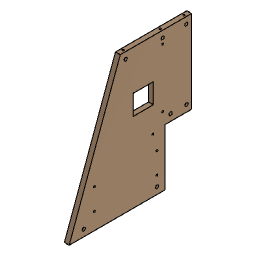
Side Panel Right (Autodesk Fusion 360 design; units mm, degrees)
Autodesk Fusion 360 part; units mm, degrees
sketch "Right" plane through (0, 0, 0) normal (1, 0, 0) x (0, 1, 0)
  line L0 (0, 0) -> (360, 0)
  line L1 (460, 212.5) -> (460, 524)
  line L2 (460, 524) -> (192, 524)
  line L3 (360, 0) -> (360, 212.5)
  line L4 (360, 212.5) -> (460, 212.5)
  line L5 (192, 524) -> (0, 0)
  line L6 (241, 374) -> (316, 374)
  line L7 (316, 374) -> (316, 299)
  line L8 (316, 299) -> (241, 299)
  line L9 (241, 299) -> (241, 374)
  line L10 (460, 499) -> (182.8397, 499) construction
  line L11 (460, 237.5) -> (316, 237.5) construction
  line L12 (360, 25) -> (9.1603, 25) construction
  line L13 (351, 524) -> (351, 250) construction
  circle A0 centre (351, 499) radius 6
  circle A1 centre (212, 499) radius 6
  circle A2 centre (440, 499) radius 6
  circle A3 centre (351, 479) radius 3.5
  circle A4 centre (351, 259) radius 3.5
  circle A5 centre (441, 237.5) radius 6
  circle A6 centre (381, 237.5) radius 6
  line L14 (330, 0) -> (330, 175) construction
  line L15 (330, 63) -> (95, 63) construction
  line L16 (95, 63) -> (95, 143) construction
  line L17 (95, 143) -> (330, 143) construction
  line L18 (330, 143) -> (330, 63) construction
  circle A7 centre (330, 63) radius 3.5
  circle A8 centre (330, 143) radius 3.5
  circle A9 centre (95, 143) radius 3.5
  circle A10 centre (95, 63) radius 3.5
  circle A11 centre (330, 25) radius 6
  circle A12 centre (55, 25) radius 6
  circle A13 centre (315, 204) radius 3.5
  dimension "d6" = 212.5
  dimension "d7" = 100
  dimension "d8" = 360
  dimension "d9" = 268
  dimension "d10" = 524
  dimension "d11" = 75
  dimension "d12" = 75
  dimension "d13" = 150
  dimension "d14" = 144
  dimension "d15" = 25
  dimension "d16" = 25
  dimension "d17" = 25
  dimension "d18" = 109
  dimension "d19" = 12
  dimension "d20" = 12
  dimension "d21" = 12
  dimension "d22" = 7
  dimension "d23" = 7
  dimension "d24" = 12
  dimension "d25" = 12
  dimension "d26" = 30
  dimension "d27" = 80
  dimension "d28" = 235
  dimension "d29" = 7
  dimension "d30" = 7
  dimension "d31" = 7
  dimension "d32" = 7
  dimension "d33" = 12
  dimension "d34" = 12
  dimension "d35" = 275
  dimension "d36" = 63
  dimension "d37" = 7
  dimension "d38" = 55
  dimension "d39" = 36
  dimension "d40" = 60
  dimension "d41" = 19
  dimension "d42" = 89
  dimension "d43" = 20
  dimension "d44" = 139
  dimension "d45" = 20
  dimension "d46" = 220
  constraint horizontal L0
  constraint vertical L1
  constraint horizontal L2
  constraint coincident L0.start L5.end
  constraint vertical L3
  constraint horizontal L4
  constraint horizontal L6
  constraint vertical L7
  constraint horizontal L8
  constraint vertical L9
  constraint coincident L1 L10.start
  constraint coincident L5 L10.end
  constraint perpendicular L1 L10
  constraint coincident L1 L11.start
  constraint perpendicular L1 L11
  constraint coincident L3 L12.start
  constraint coincident L5 L12.end
  constraint perpendicular L3 L12
  constraint coincident L2 L13.start
  constraint perpendicular L10 L13
  constraint coincident L10 A0.centre
  constraint coincident L13 A0.centre
  constraint coincident L10 A1.centre
  constraint coincident L10 A2.centre
  constraint coincident L13 A3.centre
  constraint coincident L13 A4.centre
  constraint coincident L11 A5.centre
  constraint coincident L11 A6.centre
  constraint coincident L0 L14.start
  constraint perpendicular L12 L14
  constraint horizontal L15
  constraint vertical L16
  constraint horizontal L17
  constraint vertical L18
  constraint coincident L14 L15.start
  constraint coincident L15.start L18.end
  constraint coincident L17.end L18.start
  constraint coincident L16.end L17.start
  constraint coincident L15.end L16.start
  constraint coincident L12 A11.centre
  constraint coincident L14 A11.centre
  constraint coincident L12 A12.centre
  measures "d6" distance of L0.end L3.end
  measures "d7" distance of L3.end L1.start
  measures "d8" distance of L0.start L0.end
  measures "d9" distance of L1.end L2.end
  measures "d10" distance of L0 L2
  measures "d11" distance of L6.start L6.end
  measures "d12" distance of L6.start L8.end
  measures "d13" distance of L2 L6
  measures "d14" distance of L1 L7
  measures "d15" distance of L0 L12
  measures "d16" distance of L4 L11
  measures "d17" distance of L2 L10
  measures "d18" distance of L1 L13
  measures "d19" diameter of A0
  measures "d20" diameter of A1
  measures "d21" diameter of A2
  measures "d22" diameter of A3
  measures "d23" diameter of A4
  measures "d24" diameter of A5
  measures "d25" diameter of A6
  measures "d26" distance of L3 L14
  measures "d27" distance of L15.start L17.end
  measures "d28" distance of L15.start L15.end
  measures "d29" diameter of A7
  measures "d30" diameter of A8
  measures "d31" diameter of A9
  measures "d32" diameter of A10
  measures "d33" diameter of A11
  measures "d34" diameter of A12
  measures "d35" distance of A11.centre A12.centre
  measures "d36" distance of L0 L15
  measures "d37" diameter of A13
  measures "d38" vertical distance of A4.centre A13.centre
  measures "d39" horizontal distance of A4.centre A13.centre
  measures "d40" distance of A5.centre A6.centre
  measures "d41" distance of L1 A5.centre
  measures "d42" distance of A0.centre A2.centre
  measures "d43" distance of L1 A2.centre
  measures "d44" distance of A0.centre A1.centre
  measures "d45" distance of A0.centre A3.centre
  measures "d46" distance of A3.centre A4.centre
extrude "Extrude1" add sketch "Right" along normal blind 18
sketch "Top" plane through (0, 0, 524) normal (0, 0, 1) x (-1, 0, 0)
  line L0 (0, -460) -> (0, -192)
  line L1 (0, -192) -> (-18, -192)
  line L2 (-18, -192) -> (-18, -460)
  line L3 (-18, -460) -> (0, -460)
  line L4 (-9, -192) -> (-9, -460) construction
  circle A0 centre (-9, -440) radius 3.5
  circle A1 centre (-9, -351) radius 3.5
  circle A2 centre (-9, -212) radius 3.5
  dimension "d49" = 7
  dimension "d50" = 7
  dimension "d51" = 7
  dimension "d52" = 20
  dimension "d53" = 89
  dimension "d54" = 139
  constraint midpoint L1 L4.start
  constraint midpoint L3 L4.end
  constraint coincident L4 A0.centre
  constraint coincident L4 A1.centre
  constraint coincident L4 A2.centre
  measures "d49" diameter of A0
  measures "d50" diameter of A1
  measures "d51" diameter of A2
  measures "d52" distance of L3 A0.centre
  measures "d53" distance of A0.centre A1.centre
  measures "d54" distance of A1.centre A2.centre
extrude "Extrude2" cut sketch "Top" against normal blind 35 contours A0 | A1 | A2
sketch "Sketch3" plane through (0, 0, 212.5) normal (0, 0, -1) x (1, 0, 0)
  line L0 (0, -360) -> (0, -460)
  line L1 (0, -460) -> (18, -460)
  line L2 (18, -460) -> (18, -360)
  line L3 (18, -360) -> (0, -360)
  line L4 (9, -460) -> (9, -360) construction
  circle A0 centre (9, -441) radius 3.5
  circle A1 centre (9, -381) radius 3.5
  dimension "d57" = 7
  dimension "d58" = 7
  dimension "d59" = 19
  dimension "d60" = 60
  constraint midpoint L1 L4.start
  constraint midpoint L3 L4.end
  constraint coincident L4 A0.centre
  constraint coincident L4 A1.centre
  measures "d57" diameter of A0
  measures "d58" diameter of A1
  measures "d59" distance of L1 A0.centre
  measures "d60" distance of A0.centre A1.centre
extrude "Extrude3" cut sketch "Sketch3" against normal blind 35 contours A0 | A1
sketch "Sketch4" plane through (0, 0, 0) normal (0, 0, -1) x (1, 0, 0)
  line L0 (0, 0) -> (0, -360)
  line L1 (0, -360) -> (18, -360)
  line L2 (18, -360) -> (18, 0)
  line L3 (18, 0) -> (0, 0)
  line L4 (9, 0) -> (9, -360) construction
  circle A0 centre (9, -55) radius 3.5
  circle A1 centre (9, -330) radius 3.5
  dimension "d63" = 7
  dimension "d64" = 7
  dimension "d65" = 30
  dimension "d66" = 275
  constraint midpoint L3 L4.start
  constraint midpoint L1 L4.end
  constraint coincident L4 A0.centre
  constraint coincident L4 A1.centre
  measures "d63" diameter of A0
  measures "d64" diameter of A1
  measures "d65" distance of L1 A1.centre
  measures "d66" distance of A0.centre A1.centre
extrude "Extrude4" cut sketch "Sketch4" against normal blind 35 contours A0 | A1
named bodies: "Right panel"
